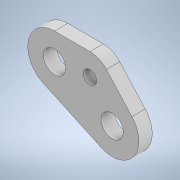
# Autodesk Inventor part: wspornik_amortyzatora
Saved by Autodesk Inventor 2020.3 (Build 243373000, 373)
## iProperties
Created: 2021-11-02
Part Number: wspornik_amortyzatora
Material: Ogólny
Document SubType Name: Modeling
Designer: patry
Density: 1 g/cm^3
Appearance: Domyślna
Author: patry
Autodesk Inventor part; units mm, degrees
ref_plane "YZ Plane" through (0, 0, 0) normal (1, 0, 0) x (0, 1, 0)
ref_plane "XZ Plane" through (0, 0, 0) normal (0, 1, 0) x (-1, 0, 0)
ref_plane "XY Plane" through (0, 0, 0) normal (0, 0, 1) x (1, 0, 0)
sketch "Szkic1" plane through (0, 0, 0) normal (0, 0, 1) x (1, 0, 0)
  circle A0 centre (0.3365, 7.2308) radius 5
  circle A1 centre (-7.6635, 6.2308) radius 6
  circle A2 centre (5.3365, 0.2308) radius 6
  line L0 (-7.6635, 12.2308) -> (0.3365, 12.2308)
  line L1 (4.0398, 10.5902) -> (9.7804, 4.2621)
  line L2 (-10.1778, 0.783) -> (2.8222, -5.217)
  point P0 (0, 0)
  dimension "d0" = 13
  dimension "d1" = 6
  dimension "d2" = 7
  dimension "d3" = 5
  dimension "d4" = 10
  dimension "d5" = 12
  dimension "d6" = 12
  constraints: 6 end point, 6 point on circle, 6 tangent, 3 centre point, 3 coincident
  measures "d0" horizontal distance of point (5.337, 0.231) point (-7.663, 6.231)
  measures "d1" vertical distance of point (5.337, 0.231) point (-7.663, 6.231)
  measures "d2" vertical distance of point (5.337, 0.231) point (0.337, 7.231)
  measures "d3" horizontal distance of point (5.337, 0.231) point (0.337, 7.231)
  measures "d4" diameter of A0
  measures "d5" diameter of A1
  measures "d6" diameter of A2
extrude "Wyciągnięcie proste1" add sketch "Szkic1" along normal blind 3
hole "Otwór1" at (5.3365, 0.2308, 0) at (-7.6635, 6.2308, 0) direction (0, 0, 1) diameter 5 end through all
hole "Otwór2" at (0.3365, 7.2308, 0) direction (0, 0, 1) diameter 3 end through all
